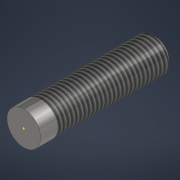
# Autodesk Inventor part: Tornillo de elevación
Saved by Autodesk Inventor 2022 (Build 260153000, 153)
## iProperties
Created: 2021-09-10
Part Number: Tornillo de elevación
Material: Stainless Steel, 440C
Document SubType Name: Modeling
Designer: Andres
Density: 7.75 g/cm^3
Appearance: Semi-Polished
Author: Andres
Autodesk Inventor part; units mm, degrees
ref_plane "YZ Plane" through (0, 0, 0) normal (1, 0, 0) x (0, 1, 0)
ref_plane "XZ Plane" through (0, 0, 0) normal (0, 1, 0) x (-1, 0, 0)
ref_plane "XY Plane" through (0, 0, 0) normal (0, 0, 1) x (1, 0, 0)
sketch "Sketch1" plane through (0, 0, 0) normal (0, 0, 1) x (1, 0, 0)
  circle A0 centre (0, 0) radius 8
  dimension "d0" = 16
  constraints: 1 centre point, 1 coincident
  measures "d0" diameter of A0
extrude "Extrusion1" add sketch "Sketch1" along normal blind 55
thread "Thread1" size "TR16x2" class "7e" standard "ISO Metric Trapezoidal Threads" length 55
sketch "Sketch2" plane through (0, 0, 55) normal (0, 0, 1) x (1, 0, 0)
  circle A0 centre (0, 0) radius 8 projected
  circle A1 centre (0, 0) radius 8 projected
  line L0 (5, 5) -> (-5, 5)
  line L1 (-5, 5) -> (-5, -5)
  line L2 (-5, -5) -> (5, -5)
  line L3 (5, -5) -> (5, 5)
  line L4 (5, 5) -> (-5, -5) construction
  line L5 (-5, 5) -> (5, -5) construction
  dimension "d11" = 10
  dimension "d12" = 10
  constraints: 12 end point, 2 midpoint, 2 parallel, 1 horizontal, 1 perpendicular
  measures "d11" distance of L2.end L1.end
  measures "d12" distance of L1.end L0.end
extrude "Extrusion2" add sketch "Sketch2" along normal blind 10 contours A0 | L3 L2 L1 L0
chamfer "Chamfer1" distance 2 angle 45 1 edges at (-8, 0, 0)
sketch "Sketch4" plane through (0, 0, 0) normal (0, 1, 0) x (-1, 0, 0)
  line L0 (8, 65) -> (-8, 65) projected
  line L1 (-8, 2) -> (8, 2) projected
  line L2 (0.1016, 57.0847) -> (0.1016, 63.0847) construction
  line L3 (1.6016, 57.0847) -> (1.6016, 63.0847)
  line L4 (-1.3984, 63.0847) -> (-1.3984, 57.0847)
  arc A0 (-1.3984, 57.0847) -> (1.6016, 57.0847) centre (0.1016, 57.0847) ccw
  arc A1 (1.6016, 63.0847) -> (-1.3984, 63.0847) centre (0.1016, 63.0847) ccw
  point P0 (0, 0)
  point P1 (0.1016, 60.0847)
  point P2 (1.5, 63)
  point P3 (-1.5, 63)
  dimension "d13" = 3
  dimension "d14" = 3
  constraints: 8 end point, 4 point on circle, 4 tangent, 2 centre point, 1 midpoint, 1 parallel, 1 vertical
  measures "d13" distance of point (0.102, 60.085) L2.end
  measures "d14" diameter of A1
extrude "Extrusion3" cut sketch "Sketch4" along normal through all
extrude "Extrusion4" add sketch "Sketch4" along normal blind 6
body "Solid1"
